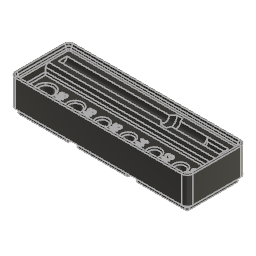
gridfinity inserts (Autodesk Fusion 360 design; units mm, degrees)
Autodesk Fusion 360 part; units mm, degrees
sketch "Sketch1" plane through (0, 0, 0) normal (0, 0, 1) x (1, 0, 0) in component "Tray"
  line L0 (0, 42) -> (42, 42)
  line L1 (42, 42) -> (42, 0)
  line L2 (42, 0) -> (0, 0)
  line L3 (0, 0) -> (0, 42)
  line L4 (0, 42) -> (42, 0) construction
  line L5 (42, 21) -> (0, 21) construction
  line L6 (42, 14.5) -> (0, 14.5)
  line L7 (42, 27.5) -> (0, 27.5)
  line L8 (27.5, 42) -> (27.5, 0)
  line L9 (14.5, 42) -> (14.5, 0)
  line L10 (14.5, 14.5) -> (0, 0) construction
  circle A0 centre (8, 8) radius 1.5
  circle A1 centre (34, 8) radius 1.5
  circle A2 centre (34, 34) radius 1.5
  circle A3 centre (8, 34) radius 1.5
  circle A4 centre (8, 8) radius 3.25
  circle A5 centre (34, 8) radius 3.25
  circle A6 centre (34, 34) radius 3.25
  circle A7 centre (8, 34) radius 3.25
  line L11 (32.5, 5.1169) -> (32.5, 10.8831)
  line L12 (35.5, 10.8831) -> (35.5, 5.1169)
  line L13 (31.1169, 6.5) -> (36.8831, 6.5)
  line L14 (36.8831, 9.5) -> (31.1169, 9.5)
  line L15 (36.8831, 32.5) -> (31.1169, 32.5)
  line L16 (35.5, 31.1169) -> (35.5, 36.8831)
  line L17 (31.1169, 35.5) -> (36.8831, 35.5)
  line L18 (32.5, 36.8831) -> (32.5, 31.1169)
  line L19 (9.5, 36.8831) -> (9.5, 31.1169)
  line L20 (10.8831, 35.5) -> (5.1169, 35.5)
  line L21 (6.5, 31.1169) -> (6.5, 36.8831)
  line L22 (5.1169, 32.5) -> (10.8831, 32.5)
  line L23 (5.1169, 9.5) -> (10.8831, 9.5)
  line L24 (6.5, 10.8831) -> (6.5, 5.1169)
  line L25 (10.8831, 6.5) -> (5.1169, 6.5)
  line L26 (9.5, 5.1169) -> (9.5, 10.8831)
  point P0 (21, 21)
  dimension "d1" = 42
  dimension "d2" = 42
  dimension "d65" = 13
  dimension "d67" = 90
  dimension "d69" = 3
  dimension "d71" = 360
  dimension "d80" = 6.5
  dimension "d85" = 8
  dimension "d185" = 360
  constraint horizontal L0
  constraint perpendicular L0 L1
  constraint parallel L0 L2
  constraint parallel L1 L3
  constraint coincident L2.end L3.start
  constraint midpoint L1 L5.start
  constraint midpoint L3 L5.end
  constraint coincident L1 L6.start
  constraint coincident L3 L6.end
  constraint perpendicular L3 L6
  constraint symmetric L5 L6.start L7.start
  constraint symmetric L5 L6.end L7.end
  constraint midpoint L4 P0
  constraint coincident L9 L10.start
  constraint coincident L6 L10.start
  constraint concentric A0 A4
  constraint coincident L10 A0.centre
  constraint coincident A5 L11.start
  constraint coincident A5 L11.end
  constraint coincident A5 L12.start
  constraint coincident A5 L12.end
  constraint coincident A5 L13.start
  constraint coincident A5 L13.end
  constraint coincident A5 L14.start
  constraint coincident A5 L14.end
  constraint tangent A1 L13
  constraint tangent A1 L14
  constraint tangent A1 L12
  constraint tangent A1 L11
  constraint horizontal L13
  constraint vertical L11
  constraint vertical L12
  constraint horizontal L14
  measures "d1" distance of L1.end L2.end
  measures "d2" distance of L0.end L1.end
  measures "d65" distance of L6 L7
  measures "d69" diameter of A0
  measures "d80" diameter of A4
  measures "d85" distance of L2 A0.centre
extrude "Extrude1" add sketch "Sketch1" along normal blind 5 contours L0 L3 L7 L9 | L0 L7 L8 L9 | L3 L6 L7 L9 | L0 L1 L7 L8 | L6 L7 L8 L9 | L2 L3 L6 L9 | L1 L6 L7 L8 | L2 L6 L8 L9 | L1 L2 L6 L8 | A0 | A0 L25 L26 | A4 L23 L25 L26 | A0 L23 L26 | A0 L23 L24 | A4 L23 L24 L26 | A0 L24 L25 | A4 L24 L25 L26 | A4 L25 L26 | A4 L23 L26 | A4 L23 L24 L25 | A4 L23 L24 | A4 L24 L25 | A1 | A1 L12 L13 | A1 L12 L14 | A5 L12 L13 L14 | A5 L11 L12 L14 | A1 L11 L14 | A1 L11 L13 | A5 L11 L12 L13 | A5 L12 L14 | A5 L12 L13 | A5 L11 L13 L14 | A5 L11 L14 | A5 L11 L13 | A2 | A2 L15 L16 | A6 L15 L16 L17 | A2 L16 L17 | A2 L17 L18 | A6 L16 L17 L18 | A2 L15 L18 | A6 L15 L16 L18 | A6 L15 L16 | A6 L16 L17 | A6 L15 L17 L18 | A6 L17 L18 | A6 L15 L18 | A3 | A3 L19 L22 | A3 L19 L20 | A7 L19 L20 L22 | A7 L19 L20 L21 | A3 L20 L21 | A3 L21 L22 | A7 L19 L21 L22 | A7 L19 L20 | A7 L19 L22 | A7 L20 L21 L22 | A7 L20 L21 | A7 L21 L22 makes body 1 in component "Tray"
ref_plane "WorkPlane1" through (21, 21, 2.5) normal (0, -1, 0) x (1, 0, 0) in component "Tray"
sketch "Sketch2" plane through (0, 21, 0) normal (0, -1, 0) x (1, 0, 0) in component "Tray"
  line L0 (42, 0) -> (0, 0)
  line L1 (0, 0) -> (0, 5)
  line L2 (3.2, 0) -> (2.4, 0.8)
  line L3 (3.2, 0) -> (0, 0) construction
  line L4 (2.4, 0.8) -> (2.4, 2.6)
  line L5 (2.4, 2.6) -> (0, 5)
  line L6 (0, 5) -> (-5.1222, 5)
  line L7 (-5.1222, 5) -> (-5.1222, -0.0937)
  line L8 (-5.1222, -0.0937) -> (0, 0)
  dimension "d39" = 45
  dimension "d40" = 45
  dimension "d41" = 0.8
  dimension "d43" = 5
  dimension "d112" = 2.4
  constraint horizontal L3
  constraint coincident L0 L2.start
  constraint perpendicular L0 L4
  constraint coincident L1 L5.end
  constraint coincident L0.end L1.start
  constraint coincident L1.end L5.end
  constraint perpendicular L1 L6
  constraint perpendicular L6 L7
  measures "d39" angle of L2 L3
  measures "d40" angle of L4 L5
  measures "d41" distance of L2.end L3
  measures "d43" distance of L3 L1.end
  measures "d112" horizontal distance of L0.end L2.end
sketch "Sketch3" plane through (0, 0, 0) normal (0, 0, -1) x (1, 0, 0)
  line L0 (42, 0) -> (0, 0)
  line L1 (0, 0) -> (0, -42)
  line L2 (0, -42) -> (42, -42)
  line L3 (42, -42) -> (42, 0)
  arc A0 (4, 0) -> (0, -4) centre (4, -4) ccw
  line L4 (0, -42) -> (42, 0) construction
  arc A1 (0, -38) -> (4, -42) centre (4, -38) ccw
  arc A2 (38, -42) -> (42, -38) centre (38, -38) ccw
  arc A3 (42, -4) -> (38, 0) centre (38, -4) ccw
  line L5 (0, -4) -> (0, -38)
  line L6 (4, -42) -> (38, -42)
  line L7 (42, -38) -> (42, -4)
  line L8 (38, 0) -> (4, 0)
  point P0 (21, -21)
  dimension "d37" = 360
  constraint coincident L1.end L2.start
  constraint coincident L0.start L3.end
  constraint midpoint L4 P0
sweep "Sweep1" cut profiles "Sketch2" path "Sketch3" along L8 A0 L5 A1 L6 A2 L7 A3 section 1 bodies 1 in component "Tray"
extrude "Extrude1'" add sketch "Sketch3" against normal up to surface (5 mm away) separate body makes body 2 in component "Blank Frame"
combine "Combine1" operation cut target body 2 tool bodies 1 keep tools in component "Blank Frame"
move_face "OffsetFaces1" offset -0.25 24 faces at (40.4, 26.6667, 3.4) (40.6565, 38.2324, 3.6667) (39.1041, 39.158, 2) (15.3333, 39.0667, 0.2667) (39.2397, 38.1085, 0.4444) (26.6667, 39.6, 1.4) (26.6667, 40.4, 3.4) (39.6, 15.3333, 1.4) (39.0667, 15.3333, 0.2667) (38.2324, 1.3435, 3.6667) (3.7676, 40.6565, 3.6667) (3.9239, 39.5982, 1.4) (3.8915, 39.2397, 0.4444) (2.4, 26.6667, 1.4) (2.9333, 15.3333, 0.2667) (1.6, 26.6667, 3.4) (1.3435, 3.7676, 3.6667) (2.4018, 3.9239, 1.4) (2.7603, 3.8915, 0.4444) (15.3333, 2.4, 1.4) (15.3333, 2.9333, 0.2667) (15.3333, 0.8, 4.2) (39.2397, 3.8915, 0.4444) (39.158, 2.8959, 1.4) on bodies 2 in component "Blank Frame"
extrude "Extrude3" [suppressed] in component "Tray"
draft "Draft1" [suppressed] in component "Tray"
pattern_linear "R-Pattern1" count 3 spacing 42 along (1, 0, 0) of bodies 1 makes body 3 at (67.3333, 15.3333, 5) makes body 4 at (109.3333, 15.3333, 5) in component "Tray"
sketch "Sketch4" plane through (0, 0, 5) normal (0, 0, 1) x (-1, 0, 0) in component "Tray"
  line L0 (-4, 0) -> (-122, 0)
  line L1 (-126, -4) -> (-126, -38)
  line L2 (-122, -42) -> (-4, -42)
  line L3 (0, -38) -> (0, -4)
  arc A0 (0, -4) -> (-4, 0) centre (-4, -4) ccw
  arc A1 (-122, 0) -> (-126, -4) centre (-122, -4) ccw
  arc A2 (-126, -38) -> (-122, -42) centre (-122, -38) ccw
  arc A3 (-4, -42) -> (0, -38) centre (-4, -38) ccw
  line L4 (-0.25, -38) -> (-0.25, -4)
  arc A4 (-0.25, -4) -> (-4, -0.25) centre (-4, -4) ccw
  line L5 (-4, -0.25) -> (-122, -0.25)
  arc A5 (-122, -0.25) -> (-125.75, -4) centre (-122, -4) ccw
  line L6 (-125.75, -4) -> (-125.75, -38)
  arc A6 (-125.75, -38) -> (-122, -41.75) centre (-122, -38) ccw
  line L7 (-122, -41.75) -> (-4, -41.75)
  arc A7 (-4, -41.75) -> (-0.25, -38) centre (-4, -38) ccw
  point P0 (-126, 0)
  point P1 (0, -42)
  dimension "d44" = 126
  dimension "d45" = 42
  dimension "d48" = 4
  dimension "d49" = 4
  dimension "d50" = 4
  dimension "d51" = 4
  dimension "d138" = -0.25
  constraint horizontal L0
  constraint vertical L1
  constraint horizontal L2
  constraint vertical L3
  constraint coincident origin L0
  constraint coincident origin L3
  constraint tangent L0 A0
  constraint tangent L3 A0
  constraint coincident P0 L0
  constraint coincident P0 L1
  constraint tangent L0 A1
  constraint tangent L1 A1
  constraint tangent L1 A2
  constraint tangent L2 A2
  constraint coincident P1 L2
  constraint coincident P1 L3
  constraint tangent L2 A3
  constraint tangent L3 A3
  measures "d44" distance of origin P0
  measures "d45" distance of origin P1
  measures "d48" radius of A0
  measures "d49" radius of A1
  measures "d50" radius of A2
  measures "d51" radius of A3
extrude "Extrude2" add sketch "Sketch4" along normal blind 16 contours L0 L1 L2 L3 A0 A1 A2 A3 | L4 A4 L5 A5 L6 A6 L7 A7 bodies 3 4 1 in component "Tray"
extrude "Extrude14" cut sketch "Sketch1" along normal blind 2.4 contours A0 | A0 L25 L26 | A4 L23 L25 L26 | A0 L23 L26 | A0 L23 L24 | A4 L23 L24 L26 | A0 L24 L25 | A4 L24 L25 L26 | A4 L25 L26 | A4 L23 L26 | A4 L23 L24 L25 | A4 L23 L24 | A4 L24 L25 | A1 | A1 L12 L13 | A1 L12 L14 | A5 L12 L13 L14 | A5 L11 L12 L14 | A1 L11 L14 | A1 L11 L13 | A5 L11 L12 L13 | A5 L12 L14 | A5 L12 L13 | A5 L11 L13 L14 | A5 L11 L14 | A5 L11 L13 | A2 | A2 L15 L16 | A6 L15 L16 L17 | A2 L16 L17 | A2 L17 L18 | A6 L16 L17 L18 | A2 L15 L18 | A6 L15 L16 L18 | A6 L15 L16 | A6 L16 L17 | A6 L15 L17 L18 | A6 L17 L18 | A6 L15 L18 | A3 | A3 L19 L22 | A3 L19 L20 | A7 L19 L20 L22 | A7 L19 L20 L21 | A3 L20 L21 | A3 L21 L22 | A7 L19 L21 L22 | A7 L19 L20 | A7 L19 L22 | A7 L20 L21 L22 | A7 L20 L21 | A7 L21 L22 bodies 3 in component "Tray"
pattern_linear "R-Pattern3" count 3 spacing 42 along (1, 0, 0) of "Extrude14" in component "Tray"
sketch "Sketch5" plane through (21, 21, 2.5) normal (0, -1, 0) x (1, 0, 0) in component "Tray"
  line L0 (-18.6, 0.1) -> (-21, 2.5)
  line L1 (101, 2.5) -> (-17, 2.5)
  line L2 (-18.6, -1.7) -> (-18.6, 0.1)
  line L3 (-17.8, -2.5) -> (-18.6, -1.7)
  line L4 (-17, 18.5) -> (-21, 18.5)
  line L5 (-17, 18.5) -> (-21, 18.5)
  line L6 (-17, 18.5) -> (101, 18.5)
  line L7 (105, 18.5) -> (101, 18.5)
  line L8 (105, 18.5) -> (101, 18.5)
  line L9 (101, 18.5) -> (-17, 18.5)
  line L10 (-18.6, 21.1) -> (-21, 23.5)
  line L11 (-18.6, 19.3) -> (-18.6, 21.1)
  line L12 (-17.8, 18.5) -> (-18.6, 19.3)
  line L13 (-21, 2.5) -> (-21, 18.5)
  line L14 (-21, 18.5) -> (-21, 2.5)
  line L15 (-17.8, 18.5) -> (-21, 18.5)
  line L16 (-21, 23.5) -> (-21, 18.5)
  line L17 (-17.9768, 18.3232) -> (-18.85, 19.1964)
  line L18 (-18.85, 19.1964) -> (-18.85, 20.9964)
  line L19 (-18.85, 20.9964) -> (-21.1768, 23.3232)
  dimension "d54" = 0
  dimension "d55" = 21
  constraint coincident L14 L4.end
  constraint perpendicular L14 L15
sweep "Sweep2" add profiles "Sketch5" along 8 edges at (126, 21, 21) (124.8284, 40.8284, 21) (63, 42, 21) (1.1716, 40.8284, 21) (0, 21, 21) (1.1716, 1.1716, 21) (63, 0, 21) (124.8284, 1.1716, 21) section 1 contours L4 L5 L15 L16 L17 L18 L19 on bodies 3 bodies 3 in component "Tray"
fillet "Fillet2" radius 0.6 8 edges at (124.8284, 1.1716, 25.6464) (126, 21, 25.6464) (124.8284, 40.8284, 25.6464) (63, 42, 25.6464) (1.1716, 40.8284, 25.6464) (0, 21, 25.6464) (1.1716, 1.1716, 25.6464) (63, 0, 25.6464) on bodies 3 in component "Tray"
sketch "Sketch6" plane through (0, 0, 21) normal (0, 0, 1) x (-1, 0, 0) in component "Tray"
  arc A0 (-4, -39.1536) -> (-2.8464, -38) centre (-4, -38) ccw
  line L0 (-2.8464, -38) -> (-2.8464, -4)
  arc A1 (-2.8464, -4) -> (-4, -2.8464) centre (-4, -4) ccw
  line L1 (-4, -2.8464) -> (-122, -2.8464)
  arc A2 (-122, -2.8464) -> (-123.1536, -4) centre (-122, -4) ccw
  line L2 (-123.1536, -4) -> (-123.1536, -38)
  arc A3 (-123.1536, -38) -> (-122, -39.1536) centre (-122, -38) ccw
  line L3 (-122, -39.1536) -> (-4, -39.1536)
  line L4 (-120.1536, -35.1536) -> (-120.1536, -31.9036)
  line L5 (-81.1536, -37.6536) -> (-85.1536, -37.6536)
  circle A4 centre (-33.7143, -12.75) radius 4.4
  line L6 (-85.1536, -37.6536) -> (-86.0635, -35.1536)
  line L7 (-81.1536, -26.1536) -> (-85.1536, -26.1536)
  line L8 (-120.1536, -28.6536) -> (-120.1536, -31.9036)
  line L9 (-5.8464, -31.9036) -> (-120.1536, -31.9036)
  circle A5 centre (-89.8679, -12.75) radius 3.65
  circle A6 centre (-108.3357, -12.75) radius 3.65
  line L10 (-86.0635, -35.1536) -> (-120.1536, -35.1536)
  line L11 (-5.8464, -34.9036) -> (-5.8464, -31.9036)
  line L12 (-86.0635, -28.6536) -> (-120.1536, -28.6536)
  circle A7 centre (-12.9964, -12.75) radius 5.15
  line L13 (-78.4036, -34.9036) -> (-81.1536, -37.6536)
  line L14 (-85.1536, -26.1536) -> (-86.0635, -28.6536)
  line L15 (-78.4036, -28.9036) -> (-81.1536, -26.1536)
  line L16 (-5.8464, -34.9036) -> (-78.4036, -34.9036)
  line L17 (-5.8464, -28.9036) -> (-78.4036, -28.9036)
  line L18 (-5.8464, -28.9036) -> (-5.8464, -31.9036)
  circle A8 centre (-71.4, -12.75) radius 3.65
  line L19 (-105.1536, -35.1536) -> (-105.1536, -28.6536)
  circle A9 centre (-52.9321, -12.75) radius 3.65
  line L20 (0, -38) -> (0, -4)
  line L21 (-126, -4) -> (-126, -38)
  line L22 (-25.1464, -2.8464) -> (-25.1464, -22.6536) construction
  line L23 (-25.1464, -22.6536) -> (-20.1464, -22.6536) construction
  line L24 (-20.1464, -22.6536) -> (-20.1464, -2.8464) construction
  line L25 (-20.1464, -2.8464) -> (-25.1464, -2.8464) construction
  line L26 (-45.1143, -2.8464) -> (-45.1143, -22.6536) construction
  line L27 (-45.1143, -22.6536) -> (-40.1143, -22.6536) construction
  line L28 (-40.1143, -22.6536) -> (-40.1143, -2.8464) construction
  line L29 (-40.1143, -2.8464) -> (-45.1143, -2.8464) construction
  line L30 (-63.5821, -2.8464) -> (-63.5821, -22.6536) construction
  line L31 (-63.5821, -22.6536) -> (-58.5821, -22.6536) construction
  line L32 (-58.5821, -22.6536) -> (-58.5821, -2.8464) construction
  line L33 (-58.5821, -2.8464) -> (-63.5821, -2.8464) construction
  line L34 (-82.05, -2.8464) -> (-82.05, -22.6536) construction
  line L35 (-82.05, -22.6536) -> (-77.05, -22.6536) construction
  line L36 (-77.05, -22.6536) -> (-77.05, -2.8464) construction
  line L37 (-77.05, -2.8464) -> (-82.05, -2.8464) construction
  line L38 (-100.5179, -2.8464) -> (-100.5179, -22.6536) construction
  line L39 (-100.5179, -22.6536) -> (-95.5179, -22.6536) construction
  line L40 (-95.5179, -22.6536) -> (-95.5179, -2.8464) construction
  line L41 (-95.5179, -2.8464) -> (-100.5179, -2.8464) construction
  line L42 (-118.9857, -2.8464) -> (-118.9857, -22.6536) construction
  line L43 (-118.9857, -22.6536) -> (-113.9857, -22.6536) construction
  line L44 (-113.9857, -22.6536) -> (-113.9857, -2.8464) construction
  line L45 (-113.9857, -2.8464) -> (-118.9857, -2.8464) construction
  line L46 (-104.6857, -12.75) -> (-93.5179, -12.75) construction
  line L47 (-86.2179, -12.75) -> (-75.05, -12.75) construction
  line L48 (-67.75, -12.75) -> (-56.5821, -12.75) construction
  line L49 (-49.2821, -12.75) -> (-38.1143, -12.75) construction
  line L50 (-29.3143, -12.75) -> (-18.1464, -12.75) construction
  line L51 (-111.9857, -12.75) -> (-123.1536, -12.75) construction
  line L52 (-7.8464, -12.75) -> (-2.8464, -12.75) construction
  line L53 (-123.1536, -22.6536) -> (-2.8464, -22.6536)
  line L54 (-12.9964, -22.6536) -> (-12.9964, -2.8464) construction
  point P0 (-12.9964, -12.75)
  dimension "d199" = 6
  dimension "d200" = 6.5
  dimension "d201" = 11.5
  dimension "d202" = 4
  dimension "d203" = 135
  dimension "d204" = 35
  dimension "d205" = 110
  dimension "d206" = 15
  dimension "d207" = 3
  dimension "d208" = 3
  dimension "d209" = 1.5
  dimension "d220" = 8.8
  dimension "d221" = 10.3
  dimension "d226" = 5
  dimension "d227" = 5
  dimension "d228" = 5
  dimension "d230" = 5
  dimension "d233" = 5
  dimension "d234" = 5
  dimension "d235" = 5
  dimension "d239" = 2
  dimension "d240" = 2
  dimension "d241" = 2
  dimension "d242" = 2
  dimension "d243" = 2
  dimension "d244" = 2
  dimension "d245" = 5
  dimension "d246" = 7.3
  dimension "d247" = 3.5
  text T0 "M8" font "Arial" height 5 align centre top in box 19.8071 x 5 at (-25.1464, -2.8464) x (0, -1) y (1, 0) spacing 1 kerned
  text T1 "M6" font "Arial" height 5 align centre top in box 19.8071 x 5 at (-45.1143, -2.8464) x (0, -1) y (1, 0) spacing 1 kerned
  text T2 "M5" font "Arial" height 5 align centre top in box 19.8071 x 5 at (-63.5821, -2.8464) x (0, -1) y (1, 0) spacing 1 kerned
  text T3 "M4" font "Arial" height 5 align centre top in box 19.8071 x 5 at (-82.05, -2.8464) x (0, -1) y (1, 0) spacing 1 kerned
  text T4 "M3" font "Arial" height 5 align centre top in box 19.8071 x 5 at (-100.5179, -2.8464) x (0, -1) y (1, 0) spacing 1 kerned
  text T5 "M2" font "Arial" height 5 align centre top in box 19.8071 x 5 at (-118.9857, -2.8464) x (0, -1) y (1, 0) spacing 1 kerned
  constraint horizontal L17
  constraint parallel L7 L17
  constraint perpendicular L17 L18
  constraint perpendicular L9 L18
  constraint perpendicular L8 L9
  constraint symmetric L11.start L17.start L9
  constraint symmetric L15.start L13.start L9
  constraint symmetric L7.start L5.start L9
  constraint symmetric L7.end L5.end L9
  constraint symmetric L6.end L12.start L9
  constraint symmetric L8.start L4.start L9
  constraint symmetric L11.end L18.end L9
  constraint coincident L19.start L10
  constraint coincident L19.end L12
  constraint perpendicular L12 L19
  constraint equal A5 A6
  constraint equal A5 A8
  constraint equal A8 A9
  constraint vertical L24
  constraint vertical L28
  constraint vertical L32
  constraint vertical L36
  constraint vertical L40
  constraint vertical L44
  constraint equal L25 L29
  constraint equal L25 L33
  constraint equal L33 L37
  constraint equal L37 L45
  constraint equal L41 L45
  constraint coincident L1
  constraint equal L24 L28
  constraint equal L28 L32
  constraint equal L32 L36
  constraint equal L36 L40
  constraint equal L40 L44
  constraint coincident A6 L46.start
  constraint coincident A5 L46.end
  constraint perpendicular L40 L46
  constraint coincident A6.centre L46
  constraint coincident A5.centre L46
  constraint coincident A8.centre L46
  constraint coincident A9.centre L46
  constraint coincident A4.centre L46
  constraint coincident P0 L46
  constraint coincident L46
  constraint coincident A5 L47.start
  constraint coincident A8 L47.end
  constraint perpendicular L36 L47
  constraint coincident A8 L48.start
  constraint coincident A9 L48.end
  constraint perpendicular L32 L48
  constraint coincident A9 L49.start
  constraint coincident A4 L49.end
  constraint perpendicular L28 L49
  constraint coincident A4 L50.start
  constraint coincident A7 L50.end
  constraint perpendicular L24 L50
  constraint coincident A6 L51.start
  constraint perpendicular L2 L51
  constraint collinear L46 L51
  constraint collinear L46 L47
  constraint collinear L47 L48
  constraint collinear L48 L49
  constraint collinear L49 L50
  constraint equal L46 L51
  constraint equal L46 L47
  constraint equal L47 L48
  constraint equal L48 L49
  constraint equal L49 L50
  constraint coincident L2 L51.end
  constraint coincident A7 L52.start
  constraint coincident L0 L52.end
  constraint perpendicular L0 L52
  constraint collinear L50 L52
  constraint coincident L2 L53.start
  constraint perpendicular L0 L53
  constraint coincident L0 L53.end
  constraint coincident L53 L54.start
  constraint coincident L1 L54.end
  constraint perpendicular L1 L54
  constraint midpoint L54 P0
  constraint coincident P0 A7.centre
  measures "d199" distance of L16 L17
  measures "d200" distance of L10 L12
  measures "d201" distance of L5 L7
  measures "d202" distance of L7.end L7.start
  measures "d203" angle of L7 L15
  measures "d204" horizontal distance of L8.start L7.end
  measures "d205" angle of L12 L14
  measures "d206" distance of L4 L19
  measures "d207" distance of L2 L4
  measures "d208" distance of L0 L11
  measures "d209" distance of L3 L5
  measures "d220" diameter of A4
  measures "d221" diameter of A7
  measures "d239" distance of L24 L50.end
  measures "d240" distance of L28 L49.end
  measures "d241" distance of L32 L48.end
  measures "d242" distance of L36 L47.end
  measures "d243" distance of L40 L46.end
  measures "d244" distance of L44 L51.start
  measures "d245" distance of L52.start L52.end
  measures "d246" diameter of A9
  measures "d247" distance of L7 L53
revolve "Revolve2" cut sketch "Sketch6" angle 360 about axis through (5.8464, 31.9036, 21) along (1, 0, 0) contours L4 L9 L10 L19 | L5 L6 L9 L10 L11 L13 L16 L19 bodies 3 in component "Tray"
extrude "Extrude13" cut sketch "Sketch6" against normal blind 3 from the near side of the face at (97.4268, 35.1495, 20.838) contours L4 L9 L10 L19 | L8 L9 L12 L19 on bodies 3 bodies 3 in component "Tray"
extrude "Extrude17" cut sketch "Sketch6" against normal blind 6 contours L0 A1 L1 A2 L2 L53 | A4 | A5 | A6 | A7 | A8 | A9 bodies 3 in component "Tray"
extrude "Extrude18" cut sketch "Sketch6" against normal blind 13.5 contours A7 bodies 3 in component "Tray"
extrude "Extrude19" cut sketch "Sketch6" against normal blind 11.8 contours A4 bodies 3 in component "Tray"
extrude "Extrude20" cut sketch "Sketch6" against normal blind 10.8 contours A9 bodies 3 in component "Tray"
extrude "Extrude21" cut sketch "Sketch6" against normal blind 11 contours A8 bodies 3 in component "Tray"
extrude "Extrude22" cut sketch "Sketch6" against normal blind 16 contours A5 | A6 bodies 3 in component "Tray"
chamfer "Chamfer2" distance 1 angle 45 6 edges at (17.7979, 10.8877, 15) (37.8165, 11.1589, 15) (56.3351, 11.4301, 15) (74.803, 11.4301, 15) (93.2708, 11.4301, 15) (111.7387, 11.4301, 15) on bodies 3 in component "Tray"
chamfer "Chamfer2" distance 2 angle 45 1 edges at (63, 22.6536, 21) on bodies 3 in component "Tray"
chamfer "Chamfer2" distance 1 angle 45 6 edges at (2.8464, 13.3268, 15) (3.1843, 3.1843, 15) (63, 2.8464, 15) (122.8157, 3.1843, 15) (123.1536, 13.3268, 15) (63, 22.6536, 15) on bodies 3 in component "Tray"
extrude "Extrude16" add sketch "Sketch6" along normal blind 0.28 from surface at -6 text T0 T1 T2 T3 T4 T5 bodies 3 in component "Tray"
component "Tray" placed x (1, 0, 0) y (0, 1, 0) z (0, 0, 1) at (0, 0, 0)
component "Blank Frame" placed x (1, 0, 0) y (0, 1, 0) z (0, 0, 1) at (0, 0, 0)
equation "d1 = slotDimension"
equation "d2 = slotDimension"
equation "d3 = nestingDepth"
equation "slotsWide = 3"
equation "slotsHigh = 1 / 2"
equation "slotsDeep = 1"
equation "slotDimension = 42 mm"
equation "nestingDepth = 5 mm"
equation "nestingRimWidth = 2.4 mm"
equation "nestingClearance = 0.25 mm"
equation "cornerFillet = 4 mm"
equation "d31 = slotsWide"
equation "d32 = slotsDeep"
equation "d33 = slotDimension"
equation "d34 = slotDimension"
equation "d38 = -slotDimension / 2"
equation "d43 = nestingDepth"
equation "d44 = slotDimension * slotsWide"
equation "d45 = slotDimension * slotsDeep"
equation "d46 = slotDimension * slotsHigh - nestingDepth"
equation "d48 = cornerFillet"
equation "d49 = cornerFillet"
equation "d50 = cornerFillet"
equation "d51 = cornerFillet"
equation "d55 = slotDimension * slotsHigh"
equation "d56 = -nestingClearance"
equation "ledStripWidth = 13 mm"
equation "ledSlotHeight = 4 mm"
equation "d65 = ledStripWidth"
equation "screwTightDiameter = 3 mm"
equation "d69 = screwTightDiameter"
equation "d72 = ledSlotHeight"
equation "magnetDiameter = 6.5 mm"
equation "magnetThiccness = 2.4 mm"
equation "d80 = magnetDiameter"
equation "d90 = -nestingClearance"
equation "wallThiccness = 1.2 mm"
equation "d112 = nestingRimWidth"
equation "d213 = magnetThiccness"
equation "d215 = slotsWide"
equation "d216 = slotsDeep"
equation "d217 = -slotDimension"
equation "d218 = slotDimension"
equation "letteringHeight = 5 mm"
equation "d236 = letteringThickness"
equation "letteringThickness = 0.28 mm"
equation "d240 = d239"
equation "d241 = d239"
equation "d242 = d239"
equation "d243 = d239"
equation "d244 = d239"
equation "d252 = 5 mm - 18.5 mm"
equation "d254 = 5 mm - 16.8 mm"
equation "d256 = 5 mm - 15.8 mm"
equation "d258 = 5 mm - 16 mm"
equation "d260 = 5 mm - 21 mm"
